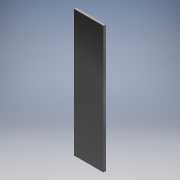
# Autodesk Inventor part: RearLeftRightTBack
Saved by Autodesk Inventor 2017 (Build 210142000, 142)
## iProperties
Created: 2016-12-13
Part Number: RearLeftRightTBack
Material: Steel, Mild
Document SubType Name: Sheet Metal
Designer: Robert.Chapman
Density: 7.85 g/cm^3
Sheet Metal Rule: Default
Appearance: Semi-Polished
Author: Robert.Chapman
Autodesk Inventor part; units mm, degrees
ref_plane "YZ Plane" through (0, 0, 0) normal (1, 0, 0) x (0, 1, 0)
ref_plane "XZ Plane" through (0, 0, 0) normal (0, 1, 0) x (-1, 0, 0)
ref_plane "XY Plane" through (0, 0, 0) normal (0, 0, 1) x (1, 0, 0)
sketch "Sketch1" plane through (0, 0, 0) normal (0, 0, 1) x (1, 0, 0)
  line L0 (-29.3687, 127) -> (29.3688, 127)
  line L1 (29.3688, 127) -> (29.3687, -127)
  line L2 (29.3687, -127) -> (-29.3688, -127)
  line L3 (-29.3688, -127) -> (-29.3687, 127)
  line L4 (-29.3687, 127) -> (29.3687, -127) construction
  line L5 (29.3688, 127) -> (-29.3688, -127) construction
  point P0 (0, 0)
  dimension "d0" = 58.7375
  dimension "d1" = 254
  measures "d0" distance of L0.start L0.end
  measures "d1" distance of L2.end L0.start
extrude "Plate1" add sketch "Sketch1" along normal blind 4.7625
equation "\"BendRadius\" = Thickness"
equation "\"BendReliefWidth\" = Thickness"
equation "\"BendReliefDepth\" = 0.5 * Thickness"
equation "\"CornerReliefSize\" = 4 * Thickness"
equation "\"MinimumRemnant\" = 2 * Thickness"
equation "\"TransitionRadius\" = BendRadius"
equation "\"JacobiRadiusSize\" = BendRadius"
equation "\"GapSize\" = Thickness"
equation "\"d2\" = BendRadius"
equation "\"Thickness\" = 4.7625"
body "Solid1"
